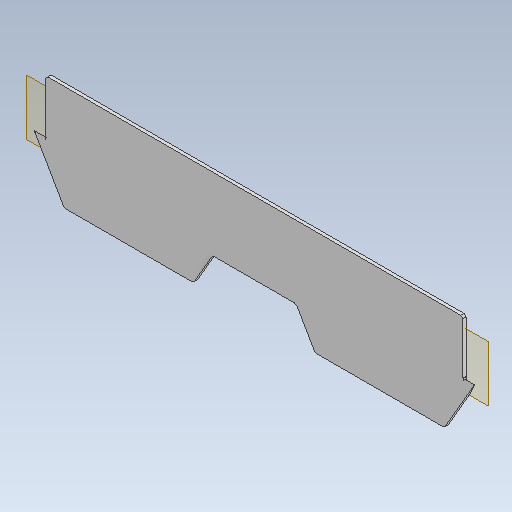
# Autodesk Inventor part: Пластина
Saved by Autodesk Inventor 2020 (Build 240168000, 168)
## iProperties
Created: 2021-05-06
Part Number: Пластина
Material: Типовые
Document SubType Name: Modeling
Designer: I_Love_U_Bogdan
Density: 1 g/cm^3
Appearance: По умолчанию
Author: I_Love_U_Bogdan
Autodesk Inventor part; units mm, degrees
ref_plane "YZ Plane" through (0, 0, 0) normal (1, 0, 0) x (0, 1, 0)
ref_plane "XZ Plane" through (0, 0, 0) normal (0, 1, 0) x (-1, 0, 0)
ref_plane "XY Plane" through (0, 0, 0) normal (0, 0, 1) x (1, 0, 0)
ref_plane "РабПлоскость1" through (0, 0, 0) normal (0, 0, 1) x (1, 0, 0)
sketch "Эскиз1" plane through (0, 0, 0) normal (0, 0, 1) x (1, 0, 0)
  line L0 (0, -90.9139) -> (0, -87.1819)
  line L1 (0, -75.9857) -> (0, -72.2537) projected
  line L2 (0, -72.2537) -> (3, -61.0575) projected
  line L3 (3, -61.0575) -> (0, -61.0575) projected
  line L4 (0, -61.0575) -> (0, -57.3255) projected
  line L5 (0, -57.3255) -> (3, -46.1293) projected
  line L6 (3, -46.1293) -> (0, -46.1293) projected
  line L7 (0, -46.1293) -> (0, -42.3973) projected
  line L8 (0, -42.3973) -> (3, -31.2011) projected
  line L9 (3, -31.2011) -> (0, -31.2011) projected
  line L10 (0, -31.2011) -> (0, -27.4691) projected
  line L11 (0, -27.4691) -> (3, -16.2729) projected
  line L12 (3, -16.2729) -> (0, -16.2729) projected
  line L13 (0, -16.2729) -> (0, -12.5409) projected
  line L14 (127.6, -12.5409) -> (0, -12.5409)
  line L15 (127.6, -57.3255) -> (124.6, -46.1293)
  line L16 (127.6, -61.0575) -> (127.6, -57.3255)
  line L17 (124.6, -61.0575) -> (127.6, -61.0575)
  line L18 (127.6, -72.2537) -> (124.6, -61.0575)
  line L19 (127.6, -75.9857) -> (127.6, -72.2537)
  line L20 (124.6, -75.9857) -> (127.6, -75.9857)
  line L21 (127.6, -87.1819) -> (124.6, -75.9857) projected
  line L22 (127.6, -90.9139) -> (127.6, -87.1819) projected
  line L23 (84.6, -94.6473) -> (84.6, -100.1704) projected
  line L24 (83.844, -94.6473) -> (84.6, -94.6473) projected
  line L25 (83.844, -94.6473) -> (84.844, -90.9152) projected
  line L26 (132.6, -90.9152) -> (84.844, -90.9152) projected
  line L27 (132.6, -90.9152) -> (134.6, -98.3793) projected
  line L28 (134.6, -98.3793) -> (134.6, 2.1319)
  line L29 (134.6, 2.1319) -> (-7, 2.1319)
  line L30 (-7, -98.3793) -> (-7, 2.1319) projected
  line L31 (-5, -90.9152) -> (-7, -98.3793) projected
  line L32 (127.6, -75.4591) -> (127.6, -90.9139) projected
  line L33 (0.2004, -110.9139) -> (127.4004, -110.9139)
  line L34 (127.4004, -110.9139) -> (127.4004, -70.9139)
  line L35 (127.4004, -70.9139) -> (0.2004, -70.9139)
  line L36 (0.2004, -70.9139) -> (0.2004, -110.9139)
  line L37 (0.2004, -110.9139) -> (127.4004, -70.9139) construction
  line L38 (127.4004, -110.9139) -> (0.2004, -70.9139) construction
  line L39 (51.0804, -92.9931) -> (38.3604, -115.0247)
  line L40 (38.3604, -115.0247) -> (12.9204, -115.0247)
  line L41 (12.9204, -115.0247) -> (0.2004, -92.9931)
  line L42 (0.2004, -70.9614) -> (63.8004, -70.9614)
  line L43 (38.3604, -70.9614) -> (51.0804, -92.9931)
  line L44 (-1, -89.7832) -> (-1, -91.3815)
  line L45 (0.2004, -92.9931) -> (5.8434, -102.7672)
  line L46 (63.8004, -70.9139) -> (63.8004, -110.9139)
  line L47 (51.0804, -92.9931) -> (63.8004, -92.9931)
  line L48 (0.2004, -92.9931) -> (-1, -90.9139)
  line L49 (5.9739, -102.9931) -> (45.3069, -102.9931)
  line L50 (-1, -90.9139) -> (0, -90.9139)
  line L51 (0, -90.9139) -> (0.2004, -90.9139)
  point P0 (0, 0)
  point P1 (63.8004, -90.9139)
  point P2 (25.6404, -92.9931)
  point P3 (5.9739, -102.9931)
  point P4 (0.3463, -70.9614)
  point P5 (0.2004, -71.5059)
  dimension "d0" = 127.6
  dimension "d1" = 127.2
  dimension "d2" = 40
  dimension "d3" = 50.88
  dimension "d4" = 0
  dimension "d5" = 1
  dimension "d6" = 25.44
  dimension "d7" = 10
  constraints: 58 end point, 7 point on line, 5 midpoint, 3 collinear, 3 parallel, 3 perpendicular, 2 horizontal, 9 other
  measures "d0" distance of L22.start L0.start
  measures "d1" distance of L35.end L34.end
  measures "d2" distance of L34.end L33.end
  measures "d3" distance of L39.start L41.end
  measures "d4" distance from line of L36 L41.end
  measures "d5" distance between parallel lines of L44 L0
  measures "d6" distance of L39.end L40.end
  measures "d7" distance from line of point (25.64, -92.993) L49
extrude "Выдавливание1" add sketch "Эскиз1" along normal blind 1 contours L36 L42 L2 | L2 L42 L43 L39 L49 L41 L36 | L36 L48 L50 L51 | L42 L46 L47 L43
chamfer "Фаска1" distance 0.5 angle 45 4 edges at (0.2004, -70.9614, 0.5) (45.3069, -102.9931, 0.5) (5.9739, -102.9931, 0.5) (51.0804, -92.9931, 0.5)
sketch "Эскиз3" plane through (0.2004, -90.9139, 0) normal (-1, 0, 0) x (0, 0, 1)
  line L0 (-2.0003, -7.4654) -> (24.9316, 93.0458) projected
  line L1 (0, 19.4526) -> (1, 19.4526) projected
  line L2 (0, 19.4526) -> (0, 0) projected
  line L3 (0, 0) -> (1, 0) projected
  line L4 (1, 19.4526) -> (1, 0) projected
  line L5 (0, 0) -> (1, 0) projected
  point P0 (0, 90.9139)
  point P1 (1, 3.7321)
extrude "Выдавливание2" add sketch "Эскиз3" along normal blind 4 contours L0 L4 L3
sketch "Эскиз4" plane through (0, 0, 1) normal (0, 0, 1) x (1, 0, 0)
  line L0 (-1, -90.9139) -> (5.7239, -102.56) projected
  line L1 (0.2004, -90.9139) -> (-1, -90.9139) projected
  line L2 (-1, -90.9139) -> (-3.1547, -87.1819)
  line L3 (0.2004, -87.1819) -> (-3.7996, -87.1819) projected
  line L4 (-1, -90.9139) -> (-3.7996, -90.9139) projected
  line L5 (-3.7996, -90.9139) -> (-3.7996, -87.1819) projected
  point P0 (0, 0)
  constraints: 2 end point, 1 collinear, 1 point on line
extrude "Выдавливание3" cut sketch "Эскиз4" against normal blind 4
sketch "Эскиз6" plane through (0, 0, 1) normal (0, 0, 1) x (1, 0, 0)
  line L0 (-3.1547, -87.1819) -> (5.7239, -102.56) projected
  line L1 (6.4739, -102.9931) -> (5.7239, -102.56) projected
  line L2 (6.4739, -102.9931) -> (44.8069, -102.9931) projected
  line L3 (45.5569, -102.56) -> (44.8069, -102.9931) projected
  line L4 (45.5569, -102.56) -> (50.8304, -93.4261) projected
  line L5 (51.5804, -92.9931) -> (50.8304, -93.4261) projected
  line L6 (51.5804, -92.9931) -> (63.8004, -92.9931) projected
  line L7 (63.8004, -92.9931) -> (63.8004, -70.9614) projected
  line L8 (63.8004, -70.9614) -> (0.7004, -70.9614) projected
  line L9 (0.2004, -71.4614) -> (0.7004, -70.9614) projected
  line L10 (0.2004, -71.4614) -> (0.2004, -87.1819) projected
  line L11 (0.2004, -87.1819) -> (-3.1547, -87.1819) projected
  line L12 (0.4004, -87.3819) -> (0.4004, -71.5442)
  line L13 (0.4004, -71.5442) -> (0.7832, -71.1614)
  line L14 (0.7832, -71.1614) -> (63.6004, -71.1614)
  line L15 (63.6004, -71.1614) -> (63.6004, -92.7931)
  line L16 (63.6004, -92.7931) -> (51.5268, -92.7931)
  line L17 (51.5268, -92.7931) -> (50.684, -93.2797)
  line L18 (50.684, -93.2797) -> (45.4105, -102.4136)
  line L19 (45.4105, -102.4136) -> (44.7533, -102.7931)
  line L20 (44.7533, -102.7931) -> (6.5275, -102.7931)
  line L21 (6.5275, -102.7931) -> (5.8703, -102.4136)
  line L22 (5.8703, -102.4136) -> (-2.8083, -87.3819)
  line L23 (-2.8083, -87.3819) -> (0.4004, -87.3819)
  line L24 (0.2004, -87.1819) -> (-3.1547, -87.1819) projected
  line L25 (0.2004, -87.1819) -> (0.4004, -87.1819)
  line L26 (0.7832, -71.1614) -> (0.9832, -70.9614)
  point P0 (0, 0)
  point P1 (0.8418, -70.9614)
  dimension "d20" = 0.2
  constraints: 28 end point, 3 point on line, 1 collinear, 11 other
  measures "d20" distance between parallel lines of L10 L12
extrude "Выдавливание5" cut sketch "Эскиз6" against normal blind 10 contours L10 L9 L8 L26 L13 L12 L25
sketch "Эскиз7" plane through (0, 0, 0) normal (0, 0, -1) x (-1, 0, 0)
  line L0 (-0.4004, -87.1819) -> (-0.4004, -71.5442) projected
  line L1 (-0.4004, -71.5442) -> (-0.9832, -70.9614) projected
  line L2 (-0.2004, -90.9139) -> (1, -90.9139) projected
  line L3 (-0.2004, -87.1819) -> (-0.2004, -90.9139) projected
  line L4 (-1.3004, -71.9614) -> (-1.3004, -88.1819)
  line L5 (-1.3004, -88.1819) -> (-1.2004, -88.1819)
  line L6 (-1.2004, -88.1819) -> (-1.2004, -91.9139)
  line L7 (-1.2004, -91.9139) -> (-0.7321, -91.9139)
  line L8 (-0.7321, -91.9139) -> (-6.4559, -101.828)
  line L9 (-6.4559, -101.828) -> (-6.7418, -101.9931)
  line L10 (-6.7418, -101.9931) -> (-44.5389, -101.9931)
  line L11 (-44.5389, -101.9931) -> (-44.8248, -101.828)
  line L12 (-44.8248, -101.828) -> (-50.0983, -92.694)
  line L13 (-50.0983, -92.694) -> (-51.3124, -91.9931)
  line L14 (-51.3124, -91.9931) -> (-62.8004, -91.9931)
  line L15 (-62.8004, -91.9931) -> (-62.8004, -71.9614)
  line L16 (-62.8004, -71.9614) -> (-1.3004, -71.9614)
  line L17 (-1.3004, -71.9614) -> (-62.8004, -81.9772) construction
  line L18 (-1.3807, -71.4679) -> (-62.8807, -81.4837)
  line L19 (-62.72, -82.4707) -> (-1.22, -72.4549)
  arc A0 (-1.22, -72.4549) -> (-1.3807, -71.4679) centre (-1.3004, -71.9614) ccw
  arc A1 (-62.8807, -81.4837) -> (-62.72, -82.4707) centre (-62.8004, -81.9772) ccw
  line L20 (-62.8004, -81.9772) -> (-1.2004, -91.9139) construction
  line L21 (-62.88, -82.4708) -> (-1.28, -92.4076)
  line L22 (-1.1207, -91.4203) -> (-62.7207, -81.4836)
  arc A2 (-62.7207, -81.4836) -> (-62.88, -82.4708) centre (-62.8004, -81.9772) ccw
  arc A3 (-1.28, -92.4076) -> (-1.1207, -91.4203) centre (-1.2004, -91.9139) ccw
  line L23 (-62.8004, -87.9931) -> (-1.2004, -87.9931) construction
  line L24 (-62.8004, -88.4931) -> (-1.2004, -88.4931)
  line L25 (-1.2004, -87.4931) -> (-62.8004, -87.4931)
  arc A4 (-62.8004, -87.4931) -> (-62.8004, -88.4931) centre (-62.8004, -87.9931) ccw
  arc A5 (-1.2004, -88.4931) -> (-1.2004, -87.4931) centre (-1.2004, -87.9931) ccw
  line L26 (-62.8004, -75.9614) -> (-1.3004, -75.9614) construction
  line L27 (-62.8004, -76.4614) -> (-1.3004, -76.4614)
  line L28 (-1.3004, -75.4614) -> (-62.8004, -75.4614)
  arc A6 (-62.8004, -75.4614) -> (-62.8004, -76.4614) centre (-62.8004, -75.9614) ccw
  arc A7 (-1.3004, -76.4614) -> (-1.3004, -75.4614) centre (-1.3004, -75.9614) ccw
  line L29 (-62.8004, -81.9772) -> (-1.3004, -81.9772) construction
  line L30 (-62.8004, -82.4772) -> (-1.3004, -82.4772)
  line L31 (-1.3004, -81.4772) -> (-62.8004, -81.4772)
  arc A8 (-62.8004, -81.4772) -> (-62.8004, -82.4772) centre (-62.8004, -81.9772) ccw
  arc A9 (-1.3004, -82.4772) -> (-1.3004, -81.4772) centre (-1.3004, -81.9772) ccw
  line L32 (-0.2004, -87.1819) -> (-0.4004, -87.1819) projected
  line L33 (-63.8004, -70.9614) -> (-0.9832, -70.9614) projected
  line L34 (-63.8004, -92.9931) -> (-63.8004, -70.9614) projected
  line L35 (-51.5804, -92.9931) -> (-63.8004, -92.9931) projected
  line L36 (-50.8304, -93.4261) -> (-51.5804, -92.9931) projected
  line L37 (-45.5569, -102.56) -> (-50.8304, -93.4261) projected
  line L38 (-44.8069, -102.9931) -> (-45.5569, -102.56) projected
  line L39 (-6.4739, -102.9931) -> (-44.8069, -102.9931) projected
  line L40 (-5.7239, -102.56) -> (-6.4739, -102.9931) projected
  line L41 (1, -90.9139) -> (-5.7239, -102.56) projected
  point P0 (0, 0)
  point P1 (-32.0504, -76.9693)
  point P2 (-32.0004, -86.9456)
  point P3 (-62.8004, -81.4706)
  point P4 (-4.411, -71.9614)
  point P5 (-0.9953, -92.37)
  point P6 (-62.8004, -82.4837)
  point P7 (-1.3004, -72.468)
  point P8 (-59.6753, -81.9749)
  point P9 (-1.2004, -91.4075)
  point P10 (-32.0004, -87.9931)
  point P11 (-32.0504, -75.9614)
  point P12 (-32.0504, -81.9772)
  point P13 (-25.9019, -75.4614)
  point P14 (-19.6807, -75.4614)
  point P15 (-1.2004, -88.4931)
  point P16 (-19.2676, -88.4931)
  point P17 (-32.0422, -76.4614)
  point P18 (-56.6197, -81.4772)
  point P19 (-1.3004, -76.4614)
  point P20 (-25.821, -76.4614)
  point P21 (-1.3004, -82.4772)
  point P22 (-56.5611, -82.4772)
  point P23 (-25.4668, -87.4931)
  point P24 (-1.3004, -87.4931)
  point P25 (-31.7461, -87.4931)
  point P26 (-25.5469, -88.4931)
  dimension "d24" = 1
  dimension "d25" = 1
  dimension "d28" = 1
  dimension "d30" = 1
  dimension "d32" = 1
  constraints: 66 end point, 20 point on circle, 20 tangent, 10 centre point, 6 midpoint, 5 parallel, 4 point on line, 3 perpendicular, 1 other
  measures "d24" diameter of A1
  measures "d25" diameter of A3
  measures "d28" diameter of A5
  measures "d30" diameter of A7
  measures "d32" diameter of A9
extrude "Выдавливание6" [suppressed]
mirror "Зеркальное отражение2" about plane through (63.8004, -92.9931, 0) normal (1, 0, 0)
